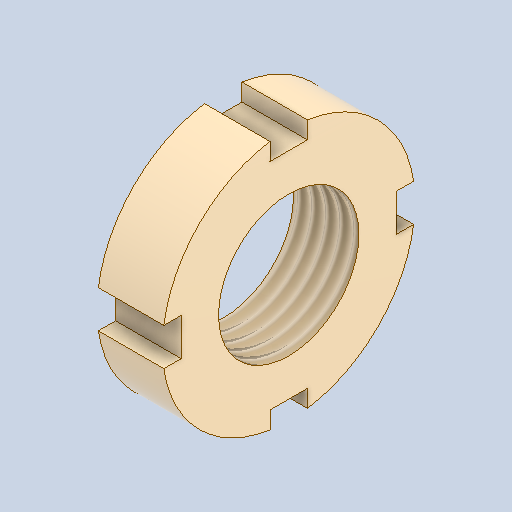
# Autodesk Inventor part: 8. LockNutM15
Saved by Autodesk Inventor 2023.2 (Build 272271030, 271C)
## iProperties
Created: 2023-03-30
Part Number: 8. LockNutM15
Material: Polyethylene, High Density
Document SubType Name: Modeling
Designer: Luis Valente
Density: 0.952 g/cm^3
Appearance: Smooth - Off-White
Author: Luis Valente
Autodesk Inventor part; units mm, degrees
ref_plane "YZ Plane" through (0, 0, 0) normal (1, 0, 0) x (0, 1, 0)
ref_plane "XZ Plane" through (0, 0, 0) normal (0, 1, 0) x (-1, 0, 0)
ref_plane "XY Plane" through (0, 0, 0) normal (0, 0, 1) x (1, 0, 0)
sketch "Sketch1" plane through (0, 0, 0) normal (1, 0, 0) x (0, 1, 0)
  circle A0 centre (0, 0) radius 13.5
  dimension "d0" = 27
  constraints: 1 centre point, 1 coincident
  measures "d0" diameter of A0
extrude "Extrusion1" add sketch "Sketch1" along normal blind 7
sketch "Sketch2" plane through (7, 0, 0) normal (1, 0, 0) x (0, 0, -1)
  circle A0 centre (0, 0) radius 7.5
  dimension "d3" = 15
  constraints: 1 centre point, 1 coincident
  measures "d3" diameter of A0
extrude "Extrusion2" cut sketch "Sketch2" against normal blind 7
thread "Thread1" size "M15x1.5" class "6H" standard "ISO Metric profile" length 13
sketch "Sketch3" plane through (7, 0, 0) normal (1, 0, 0) x (0, 0, -1)
  circle A0 centre (0, 0) radius 13.5 projected
  line L0 (0, 13.5) -> (0, 11.5)
  line L1 (0, 11.5) -> (-2, 11.5)
  line L2 (-2, 11.5) -> (2, 11.5)
  line L3 (2, 11.5) -> (2, 14.5713)
  line L4 (2, 14.5713) -> (-2, 14.5713)
  line L5 (-2, 14.5713) -> (-2, 11.5)
  line L6 (-13.5, 0) -> (-11.5, 0)
  line L7 (-11.5, 0) -> (-11.5, -2)
  line L8 (-11.5, -2) -> (-11.5, 2)
  line L9 (-11.5, 2) -> (-14.5713, 2)
  line L10 (-14.5713, 2) -> (-14.5713, -2)
  line L11 (-14.5713, -2) -> (-11.5, -2)
  line L12 (0, -13.5) -> (0, -11.5)
  line L13 (0, -11.5) -> (2, -11.5)
  line L14 (2, -11.5) -> (-2, -11.5)
  line L15 (-2, -11.5) -> (-2, -14.5713)
  line L16 (-2, -14.5713) -> (2, -14.5713)
  line L17 (2, -14.5713) -> (2, -11.5)
  line L18 (13.5, 0) -> (11.5, 0)
  line L19 (11.5, 0) -> (11.5, 2)
  line L20 (11.5, 2) -> (11.5, -2)
  line L21 (11.5, -2) -> (14.5713, -2)
  line L22 (14.5713, -2) -> (14.5713, 2)
  line L23 (14.5713, 2) -> (11.5, 2)
  dimension "d8" = 2
  dimension "d9" = 2
  dimension "d10" = 4
  dimension "d13" = 360
  constraints: 48 end point, 4 point on line, 3 perpendicular, 1 horizontal, 1 vertical, 1 vertical alignment, 50 other
  measures "d8" distance of L0.start L0.end
  measures "d9" distance of L0.end L1.end
  measures "d10" distance of L1.end L2.end
extrude "Extrusion3" cut sketch "Sketch3" against normal blind 7 contours L18 L19 L23 A0 | A0 L23 L22 L21 | A0 L21 L20 L18 | L3 L2 L0 A0 | A0 L5 L4 L3 | L17 L16 L15 A0 | A0 L12 L13 L17 | L0 L1 L5 A0 | A0 L15 L14 L12 | L9 L8 L6 A0 | A0 L11 L10 L9 | A0 L6 L7 L11
body "Solid1"
